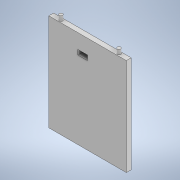
# Autodesk Inventor part: expo4
Saved by Autodesk Inventor 2020 (Build 240168000, 168)
## iProperties
Created: 2020-02-18
Part Number: expo4
Material: Generic
Document SubType Name: Modeling
Designer: Aryan
Density: 1 g/cm^3
Appearance: Default
Author: Aryan
Autodesk Inventor part; units mm, degrees
ref_plane "YZ Plane" through (0, 0, 0) normal (1, 0, 0) x (0, 1, 0)
ref_plane "XZ Plane" through (0, 0, 0) normal (0, 1, 0) x (-1, 0, 0)
ref_plane "XY Plane" through (0, 0, 0) normal (0, 0, 1) x (1, 0, 0)
sketch "Sketch1" plane through (0, 0, 0) normal (0, 1, 0) x (-1, 0, 0)
  line L0 (0, 0) -> (-80, 0)
  line L1 (-80, 0) -> (-80, -5)
  line L2 (-80, -5) -> (0, -5)
  line L3 (0, -5) -> (0, 0)
  dimension "d0" = 80
  dimension "d1" = 5
  constraints: 8 end point, 2 parallel, 1 horizontal, 1 perpendicular
  measures "d0" distance of L2.end L1.end
  measures "d1" distance of L1.end L0.end
extrude "Extrusion1" add sketch "Sketch1" along normal blind 100
sketch "Sketch2" plane through (0, 100, 0) normal (0, 1, 0) x (1, 0, 0)
  line L0 (0, 0) -> (10, 0)
  line L1 (10, 0) -> (10, 2.5)
  line L2 (10, 2.5) -> (0, 2.5)
  line L3 (0, 2.5) -> (0, 0)
  circle A0 centre (10, 2.5) radius 1.75
  dimension "d4" = 10
  dimension "d5" = 2.5
  dimension "d6" = 3.5
  constraints: 8 end point, 2 parallel, 1 centre point, 1 coincident, 1 horizontal, 1 perpendicular
  measures "d4" distance of L2.end L1.end
  measures "d5" distance of L1.end L0.end
  measures "d6" diameter of A0
extrude "Extrusion2" add sketch "Sketch2" along normal blind 5 contours A0 L2 L1 | L1 L2 A0
sketch "Sketch3" plane through (0, 100, 0) normal (0, 1, 0) x (1, 0, 0)
  line L0 (80, 5) -> (0, 5) projected
  line L1 (80, 5) -> (70, 5)
  line L2 (70, 5) -> (70, 2.5)
  line L3 (70, 2.5) -> (80, 2.5)
  line L4 (80, 2.5) -> (80, 5)
  circle A0 centre (70, 2.5) radius 1.75
  point P0 (0, 0)
  dimension "d9" = 10
  dimension "d10" = 2.5
  dimension "d11" = 3.5
  constraints: 8 end point, 2 parallel, 1 centre point, 1 coincident, 1 horizontal, 1 perpendicular
  measures "d9" distance of L3.end L2.end
  measures "d10" distance of L2.end L1.end
  measures "d11" diameter of A0
extrude "Extrusion3" add sketch "Sketch3" along normal blind 5 contours A0 L3 L2 | L2 L3 A0
sketch "Sketch4" plane through (0, 0, 0) normal (0, 0, 1) x (1, 0, 0)
  line L0 (0, 0) -> (80, 0) projected
  line L1 (80, 0) -> (40, 0)
  line L2 (40, 0) -> (40, 80)
  line L3 (40, 80) -> (80, 80)
  line L4 (80, 80) -> (80, 0)
  line L5 (40, 80) -> (30, 80)
  line L6 (30, 80) -> (30, 85)
  line L7 (30, 85) -> (40, 85)
  line L8 (40, 85) -> (40, 80)
  dimension "d14" = 40
  dimension "d15" = 80
  dimension "d16" = 10
  dimension "d17" = 5
  constraints: 16 end point, 4 parallel, 2 horizontal, 2 perpendicular
  measures "d14" distance of L2.end L3.end
  measures "d15" distance of L1.end L2.end
  measures "d16" distance of L6.end L7.end
  measures "d17" distance of L5.end L6.end
extrude "Extrusion4" cut sketch "Sketch4" against normal blind 10 contours L5 L6 L7 L8
body "Solid1"
